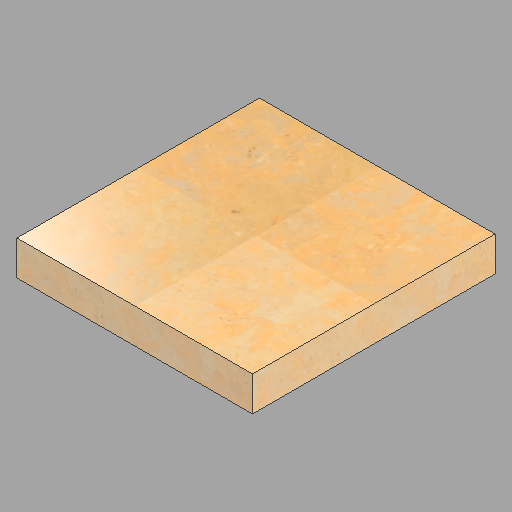
# Autodesk Inventor part: A - Split face veneer - 10
Saved by Autodesk Inventor 2022.2 (Build 262287010, 287A)
## iProperties
RuleStatus: InUse
Created: 2022-03-23
Part Number: A - Split face veneer - 10
Material: Granite, Cut, Polished
Document SubType Name: Modeling
Designer: awelt
Mass: 32907.3 g
Surface Area: 4951.6 cm^2
Volume: 12187.9 cm^3
Density: 2.7 g/cm^3
Appearance: Amber Select
AfterDocSave0: Convert in3 volume to ft3
in3 to ft3: 0.43
TEST: 0.43
Author: awelt
Autodesk Inventor part; units mm, degrees
ref_plane "YZ Plane" through (0, 0, 0) normal (1, 0, 0) x (0, 1, 0)
ref_plane "XZ Plane" through (0, 0, 0) normal (0, 1, 0) x (-1, 0, 0)
ref_plane "XY Plane" through (0, 0, 0) normal (0, 0, 1) x (1, 0, 0)
sketch "Sketch1" plane through (0, 0, 0) normal (0, 1, 0) x (-1, 0, 0)
  line L0 (215.9, -222.25) -> (-215.9, -222.25)
  line L1 (-215.9, -222.25) -> (-215.9, 222.25)
  line L2 (-215.9, 222.25) -> (215.9, 222.25)
  line L3 (215.9, 222.25) -> (215.9, -222.25)
  line L4 (215.9, -222.25) -> (-215.9, 222.25) construction
  line L5 (-215.9, -222.25) -> (215.9, 222.25) construction
  point P0 (0, 0)
  dimension "d0" = 431.8
  dimension "d1" = 444.5
  constraints: 12 end point, 2 midpoint, 2 parallel, 1 horizontal, 1 perpendicular
  measures "d0" distance of L1.end L2.end
  measures "d1" distance of L0.end L1.end
extrude "Extrusion1" add sketch "Sketch1" along normal blind 63.5
body "Solid1"
